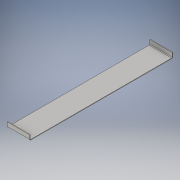
# Autodesk Inventor part: Side Gurad
Saved by Autodesk Inventor 2016 (Build 200138000, 138)
## iProperties
Created: 2018-05-16
Part Number: Side Gurad
Material: Generic
Document SubType Name: Sheet Metal
Designer: Kade
Density: 1 g/cm^3
Sheet Metal Rule: Default
Appearance: Default
Mass: 252.213 g
Surface Area: 1644.11 cm^2
Volume: 252.213 cm^3
Author: Kade
Autodesk Inventor part; units mm, degrees
ref_plane "YZ Plane" through (0, 0, 0) normal (1, 0, 0) x (0, 1, 0)
ref_plane "XZ Plane" through (0, 0, 0) normal (0, 1, 0) x (-1, 0, 0)
ref_plane "XY Plane" through (0, 0, 0) normal (0, 0, 1) x (1, 0, 0)
sketch "Sketch1" plane through (0, 0, 0) normal (0, 1, 0) x (-1, 0, 0)
  line L0 (-56.1975, 358.902) -> (56.1975, 358.902)
  line L1 (56.1975, 358.902) -> (56.1975, -358.902)
  line L2 (56.1975, -358.902) -> (-56.1975, -358.902)
  line L3 (-56.1975, -358.902) -> (-56.1975, 358.902)
  line L4 (-56.1975, 358.902) -> (56.1975, -358.902) construction
  line L5 (56.1975, 358.902) -> (-56.1975, -358.902) construction
  point P0 (0, 0)
  dimension "d0" = 112.395
  dimension "d1" = 717.804
  measures "d0" distance of L1.end L2.end
  measures "d1" distance of L0.end L1.end
extrude "Plate1" add sketch "Sketch1" along normal blind 3.048
sketch "Sketch2" plane through (56.1975, 0, 355.854) normal (0, 0, 1) x (1, 0, 0)
  line L0 (-112.395, 0) -> (0, 0)
  line L1 (0, 0) -> (0, 25.4)
  line L2 (0, 25.4) -> (-112.395, 25.4)
  line L3 (-112.395, 25.4) -> (-112.395, 0)
  constraints: 6 end point, 1 horizontal, 1 perpendicular, 1 vertical
edge flange "Flange1" height 25.4 angle 90 thickness 3.048 bend radius 3.048 thickness toward (0, 0, 1) relief straight relief width 3.048 relief depth 1.524 corner gap 3.048 corner form 0 edges at (0, 3.048, 358.902) (0, 3.048, -358.902) wall of the first edge with corners at (-56.1975, 0, 355.854) (56.1975, 0, 355.854) (56.1975, 25.4, 355.854) (-56.1975, 25.4, 355.854)
bend "Bend1"
corner "Corner1"
equation "\"d5\" = BendReliefWidth"
equation "\"d6\" = BendReliefDepth"
equation "\"d7\" = MinimumRemnant"
equation "\"d8\" = BendRadius"
equation "\"d11\" = BendRadius"
equation "\"d12\" = CornerReliefSize"
equation "\"d13\" = GapSize"
equation "\"d14\" = JacobiRadiusSize"
equation "\"BendRadius\" = Thickness"
equation "\"BendReliefWidth\" = Thickness"
equation "\"BendReliefDepth\" = 0.5 * Thickness"
equation "\"CornerReliefSize\" = 4 * Thickness"
equation "\"MinimumRemnant\" = 2 * Thickness"
equation "\"TransitionRadius\" = BendRadius"
equation "\"JacobiRadiusSize\" = Thickness"
equation "\"GapSize\" = Thickness"
equation "\"d4\" = BendRadius"
equation "\"Thickness\" = 3.048"
body "Solid2"
